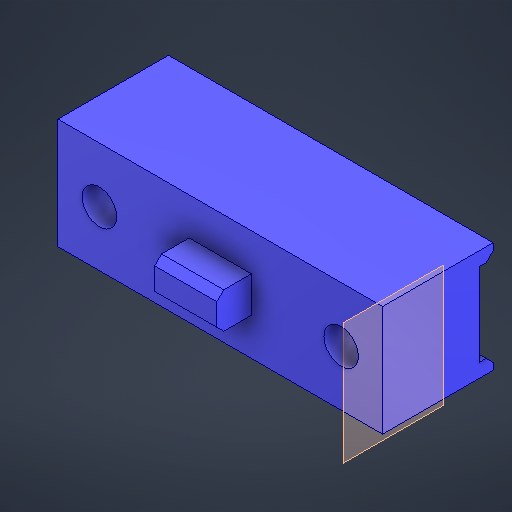
# Autodesk Inventor part: Bearing Spacer_1.5mmUP
Saved by Autodesk Inventor 2026.2 (Build 302298010, 298A)
## iProperties
Created: 2026-06-01
Part Number: Bearing Spacer_1.5mmUP
Material: 일반
Document SubType Name: Modeling
Designer: dalbi
Density: 1 g/cm^3
Appearance: 기본값
Author: dalbi
Autodesk Inventor part; units mm, degrees
ref_plane "YZ Plane" through (0, 0, 0) normal (1, 0, 0) x (0, 1, 0)
ref_plane "XZ Plane" through (0, 0, 0) normal (0, 1, 0) x (-1, 0, 0)
ref_plane "XY Plane" through (0, 0, 0) normal (0, 0, 1) x (1, 0, 0)
ref_plane "작업 평면1" through (23.5, -8, -2) normal (1, 0, 0) x (0, 0, -1)
sketch "스케치1" plane through (23.5, -8, -2) normal (1, 0, 0) x (0, 0, -1)
  line L0 (0, 16) -> (-8.15, 16) projected
  line L1 (-8.15, 16) -> (-8.15, 10.6) projected
  line L2 (-8.15, 10.6) -> (-12.15, 10.6) projected
  line L3 (-13.15, 9.6) -> (-12.15, 10.6) projected
  line L4 (-13.15, 9.6) -> (-13.15, 6.4) projected
  line L5 (-12.15, 5.4) -> (-13.15, 6.4) projected
  line L6 (-12.15, 5.4) -> (-8.15, 5.4) projected
  line L7 (-8.15, 5.4) -> (-8.15, 0) projected
  line L8 (-8.15, 0) -> (0, 0) projected
  line L9 (0, 16) -> (7.85, 16)
  line L10 (7.85, 16) -> (7.85, 15)
  line L11 (7.85, 15) -> (6.85, 14)
  line L12 (5.85, 14) -> (5.85, 2)
  line L13 (5.85, 14) -> (6.85, 14)
  line L14 (0, 0) -> (7.85, 0)
  line L15 (7.85, 0) -> (7.85, 1)
  line L16 (7.85, 1) -> (6.85, 2)
  line L17 (5.85, 2) -> (6.85, 2)
  line L18 (0, 16) -> (-8.15, 16)
  line L19 (-8.15, 10.6) -> (-12.15, 10.6) projected
  line L20 (-8.15, 10.6) -> (-12.15, 10.6)
  line L21 (-12.15, 10.6) -> (-13.15, 9.6)
  line L22 (-13.15, 6.4) -> (-12.15, 5.4)
  point P0 (-2, 8)
  dimension "d1" = 7.85
  constraints: 26 end point, 3 horizontal, 2 collinear, 2 perpendicular, 1 vertical
  measures "d1" distance of L0.start L9.end
sketch "스케치2" plane through (-23.5, 8, 6.15) normal (0, 0, 1) x (1, 0, 0)
  arc A0 (7.9209, -9.6) -> (7.9209, -6.4) centre (6, -8) ccw projected
  line L0 (39.0791, -9.6) -> (7.9209, -9.6) projected
  circle A1 centre (6, -8) radius 2.5
  circle A2 centre (41, -8) radius 2.5 projected
  circle A3 centre (41, -8) radius 2.5
  point P0 (23.5, -8)
  point P1 (7.9209, -6.4)
  constraints: 2 coincident, 1 centre point, 4 other
extrude "돌출1" add sketch "스케치1" against normal up to surface (47 mm away)
extrude "돌출2" cut sketch "스케치2" along normal mid plane 50
sketch "스케치3" plane through (-15.5791, 1.6, 11.15) normal (0, 0, 1) x (1, 0, 0)
  line L0 (15.5791, -14.4593) -> (15.5791, 15.5737)
  line L1 (-7.9209, 4.4) -> (-7.9209, -7.6) projected
  line L2 (-7.9209, 4.4) -> (11.0791, 4.4)
  line L3 (11.0791, 4.4) -> (11.0791, -7.6)
  line L4 (11.0791, -7.6) -> (-7.9209, -7.6)
  line L5 (-7.9209, -7.6) -> (-7.9209, 4.4)
  line L6 (39.0791, 4.4) -> (39.0791, -7.6)
  line L7 (39.0791, 4.4) -> (20.0791, 4.4)
  line L8 (20.0791, 4.4) -> (20.0791, -7.6)
  line L9 (20.0791, -7.6) -> (39.0791, -7.6)
  line L10 (39.0791, -7.6) -> (39.0791, 4.4)
  point P0 (15.5791, -1.6)
  dimension "d9" = 19
  constraints: 20 end point, 5 symmetric about line, 2 parallel, 1 horizontal, 1 perpendicular, 1 vertical
  measures "d9" distance of L1.start L2.end
extrude "돌출3" cut sketch "스케치3" against normal up to surface (5 mm away)
